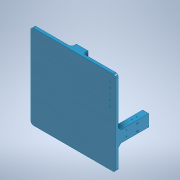
# Autodesk Inventor part: frame
Saved by Autodesk Inventor 2020 (Build 240168000, 168)
## iProperties
Created: 2026-07-10
Part Number: frame
Material: Iron, Gray
Document SubType Name: Modeling
Designer: drago
Density: 7.15 g/cm^3
Appearance: Sky Blue Dark
Author: drago
Autodesk Inventor part; units mm, degrees
ref_plane "YZ Plane" through (0, 0, 0) normal (1, 0, 0) x (0, 1, 0)
ref_plane "XZ Plane" through (0, 0, 0) normal (0, 1, 0) x (-1, 0, 0)
ref_plane "XY Plane" through (0, 0, 0) normal (0, 0, 1) x (1, 0, 0)
sketch "Sketch1" plane through (0, 0, 0) normal (0, 0, 1) x (1, 0, 0)
  line L0 (155, 0) -> (155, -21.8)
  line L1 (162, -21.8) -> (166.7129, -21.8)
  line L2 (155, 0) -> (166.3149, 0)
  line L3 (166.3149, 0) -> (166.3149, -21.8)
  line L4 (166.3149, -21.8) -> (155, -21.8)
  line L5 (155, -21.8) -> (155, 0)
  circle A0 centre (160, -5) radius 1
  circle A1 centre (160, -5) radius 1
  circle A2 centre (160, -16.8) radius 1
  circle A3 centre (160, -16.8) radius 1
  circle A4 centre (20, -16.8) radius 1
  circle A5 centre (20, -16.8) radius 1
  circle A6 centre (20, -5) radius 1
  circle A7 centre (20, -5) radius 1
  line L6 (24, 0) -> (24, -21.8)
  line L7 (8, 0) -> (8.5, 0)
  line L8 (8.5, 0) -> (8.5, -21.8)
  line L9 (24, 0) -> (8.5, 0)
  line L10 (8.5, 0) -> (8.5, -21.8)
  line L11 (8.5, -21.8) -> (24, -21.8)
  line L12 (24, -21.8) -> (24, 0)
  point P0 (0, 0)
  constraints: 26 end point, 8 centre point, 4 coincident, 4 parallel, 3 horizontal, 3 perpendicular, 1 point on line
extrude "Extrusion1" add sketch "Sketch1" against normal blind 10
extrude "Extrusion2" add sketch "Sketch1" along normal blind 37.5 contours L2 L3 L1 L4 L0 | A0 | A2 | A4 | A6 | L6 L11 L8 L9
sketch "Sketch2" plane through (166.3149, -21.8, -10) normal (1, 0, 0) x (0, 0, -1)
  line L0 (-47.5, 21.8) -> (-47.5, 0) projected
  line L1 (0, 21.8) -> (-47.5, 21.8) projected
  line L2 (0, 0) -> (-47.5, 0) projected
  circle A0 centre (-21.95, 3.95) radius 1.4
  circle A1 centre (-21.95, 16.35) radius 1.4
  point P0 (-10, 21.8)
  constraints: 2 centre point
extrude "Extrusion3" cut sketch "Sketch2" against normal blind 500
sketch "Sketch3" plane through (0, 0, 37.5) normal (0, 0, 1) x (1, 0, 0)
  line L0 (24, -21.8) -> (24, 0) projected
  circle A0 centre (84.1, -53.8) radius 0.9
  circle A1 centre (95.9, -53.8) radius 0.9
  circle A2 centre (95.9, 86.2) radius 0.9
  circle A3 centre (84.1, 86.2) radius 0.9
  line L1 (95.9, 92.2) -> (8.5, 92.2)
  line L2 (8.5, 92.2) -> (8.5, -64.8)
  line L3 (8.5, -64.8) -> (95.9, -64.8)
  line L4 (95.9, -64.8) -> (166.3149, -64.8)
  line L5 (166.3149, -64.8) -> (166.3149, 92.2)
  line L6 (166.3149, 92.2) -> (95.9, 92.2)
  line L7 (100.9, -42.8) -> (79.1, -42.8)
  line L8 (79.1, -42.8) -> (79.1, -64.8)
  line L9 (79.1, -64.8) -> (100.9, -64.8)
  line L10 (100.9, -64.8) -> (100.9, -42.8)
  line L11 (100.9, 80.2) -> (79.1, 80.2)
  line L12 (79.1, 80.2) -> (79.1, 92.2)
  line L13 (79.1, 92.2) -> (100.9, 92.2)
  line L14 (100.9, 92.2) -> (100.9, 80.2)
  line L15 (166.3149, 0) -> (166.3149, -21.8) projected
  line L16 (155, -21.8) -> (155, 0) projected
  line L17 (166.3149, -21.8) -> (155, -21.8)
  line L18 (155, -21.8) -> (155, 0)
  line L19 (155, 0) -> (166.3149, 0)
  line L20 (166.3149, 0) -> (166.3149, -21.8)
  line L21 (8.5, -21.8) -> (24, -21.8) projected
  line L22 (24, 0) -> (8.5, 0) projected
  line L23 (24, -21.8) -> (8.5, -21.8)
  line L24 (8.5, -21.8) -> (8.5, 0)
  line L25 (8.5, 0) -> (24, 0)
  line L26 (24, 0) -> (24, -21.8)
  point P0 (0, 0)
  point P1 (90, -53.8)
  constraints: 44 end point, 10 parallel, 6 horizontal, 6 perpendicular, 4 centre point, 2 point on line
extrude "Extrusion4" add sketch "Sketch3" along normal blind 15 contours L21 L2 L22 L0 | L0 L22 L2 L1 L12 L11 L14 L6 L5 L19 L16 L17 L4 L10 L7 L8 L3 L21 | L8 L7 L10 L4 L3 | L1 L6 L14 L11 L12 | L17 L16 L19 L5 | A0 | A1 | A2 | A3
extrude "Extrusion5" cut sketch "Sketch3" along normal blind 10 contours L0 L22 L2 L1 L12 L11 L14 L6 L5 L19 L16 L17 L4 L10 L7 L8 L3 L21 | A0 | A1 | A2 | A3
chamfer "Chamfer1" distance 5 angle 45 6 edges at (160.6575, 0, 47.5) (155, -10.9, 47.5) (160.6575, -21.8, 47.5) (16.25, 0, 47.5) (24, -10.9, 47.5) (16.25, -21.8, 47.5)
chamfer "Chamfer2" distance 3 angle 45 6 edges at (79.1, -53.8, 47.5) (90, -42.8, 47.5) (100.9, -53.8, 47.5) (90, 80.2, 47.5) (79.1, 86.2, 47.5) (100.9, 86.2, 47.5)
fillet "Fillet1" radius 5 4 edges at (8.5, 92.2, 50) (166.3149, 92.2, 50) (166.3149, -64.8, 50) (8.5, -64.8, 50)
fillet "Fillet2" radius 1 16 edges at (155, -10.9, -10) (160.6575, 0, -10) (166.3149, -10.9, -10) (160.6575, -21.8, -10) (16.25, -21.8, -10) (24, -10.9, -10) (8.5, -10.9, -10) (16.25, 0, -10) (79.1, -53.8, 37.5) (90, -64.8, 37.5) (100.9, -53.8, 37.5) (90, -42.8, 37.5) (90, 80.2, 37.5) (79.1, 86.2, 37.5) (100.9, 86.2, 37.5) (90, 92.2, 37.5)
chamfer "Chamfer3" distance 0.5 angle 45 8 edges at (95, 86.2, 37.5) (83.2, 86.2, 37.5) (19, -16.8, -10) (19, -5, -10) (95, -53.8, 37.5) (83.2, -53.8, 37.5) (159, -16.8, -10) (159, -5, -10)
sketch "Sketch4" plane through (8.5, 0, 42.5) normal (0, 1, 0) x (1, 0, 0)
  circle A0 centre (7.75, 26.15) radius 0.9
  circle A1 centre (7.75, 34.95) radius 0.9
  circle A2 centre (152.1575, 26.15) radius 0.9
  circle A3 centre (152.1575, 34.95) radius 0.9
  point P0 (-8.5, 42.5)
  dimension "d43" = 1.8
  dimension "d44" = 1.8
  constraints: 4 centre point
  measures "d43" diameter of A0
  measures "d44" diameter of A1
extrude "Extrusion6" cut sketch "Sketch4" against normal blind 10
sketch "Sketch5" plane through (0, 0, 47.5) normal (0, 0, -1) x (-1, 0, 0)
  circle A0 centre (-18.5, 25) radius 1.4
  circle A1 centre (-58.5, 65) radius 1.4
  circle A2 centre (-58.5, 65) radius 4.5
  circle A3 centre (-18.5, 25) radius 4.5
  point P0 (0, 0)
  point P1 (-8.5, 5)
  constraints: 4 centre point, 2 coincident
extrude "Extrusion7" add sketch "Sketch5" along normal blind 15
chamfer "Chamfer4" distance 0.5 angle 45 4 edges at (59.9, 65, 32.5) (63, 65, 32.5) (19.9, 25, 32.5) (23, 25, 32.5)
chamfer "Chamfer5" distance 1 angle 45 2 edges at (23, 25, 47.5) (63, 65, 47.5)
sketch "Sketch6" plane through (0, 0, 47.5) normal (0, 0, -1) x (-1, 0, 0)
  arc A0 (-161.3149, 92.2) -> (-166.3149, 87.2) centre (-161.3149, 87.2) ccw projected
  line L0 (-166.3149, 87.2) -> (-156.3149, 87.2)
  line L1 (-156.3149, 87.2) -> (-156.3149, 77.2)
  circle A1 centre (-156.3149, 77.2) radius 0.9
  circle A2 centre (-156.3149, 67.2) radius 0.9
  circle A3 centre (-156.3149, 57.2) radius 0.9
  circle A4 centre (-156.3149, 47.2) radius 0.9
  circle A5 centre (-156.3149, 37.2) radius 0.9
  point P0 (0, 0)
  dimension "d65" = 10
  dimension "d70" = 1.8
  constraints: 5 centre point, 4 end point, 1 coincident, 1 horizontal, 1 perpendicular
  measures "d65" distance of L0.end L1.end
  measures "d70" diameter of A1
extrude "Extrusion8" cut sketch "Sketch6" against normal blind 10
sketch "Sketch7" plane through (166.3149, -59.8, 52.5) normal (1, 0, 0) x (0, 0, -1)
  line L0 (61.5, 59.8) -> (10, 59.8) projected
  line L1 (10, 59.8) -> (20, 59.8)
  line L2 (61.5, 38) -> (10, 38) projected
  circle A0 centre (20, 54.35) radius 0.9
  circle A1 centre (20, 43.45) radius 0.9
  point P0 (52.5, 59.8)
  dimension "d73" = 10
  dimension "d74" = 1.8
  constraints: 2 centre point, 2 end point, 1 point on line
  measures "d73" distance of L0.end L1.end
  measures "d74" diameter of A0
extrude "Extrusion9" cut sketch "Sketch7" against normal blind 10
body "Solid1"
